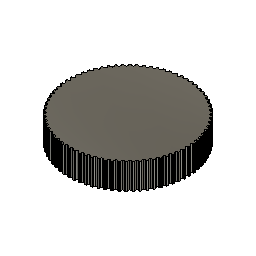
gear_74z (Autodesk Fusion 360 design; units mm, degrees)
Autodesk Fusion 360 part; units mm, degrees
sketch "Sketch1" plane through (0, 0, 0) normal (0, 0, 1) x (1, 0, 0) in component "gt2 pulley"
  circle A0 centre (0, 0) radius 23.5549 construction
  circle A1 centre (0, 0) radius 22.5509 construction
  line L0 (0, 0) -> (0, 23.5549) construction
  line L1 (0, 0) -> (0.9997, 23.5337) construction
  line L2 (0, 0) -> (1.4052, 23.513) construction
  circle A2 centre (0, 0) radius 23.3009 construction
  arc A3 (0.3946, 23.164) -> (0.47, 22.8677) centre (1.3901, 23.2594) ccw
  circle A4 centre (0, 0) radius 23.1509 construction
  arc A5 (0.2469, 23.2996) -> (0, 23.3009) centre (0, 0) ccw
  arc A6 (0.3946, 23.164) -> (0.2469, 23.2996) centre (0.2453, 23.1496) ccw
  arc A7 (0.47, 22.8677) -> (0.9571, 22.5306) centre (0.9806, 23.0851) ccw
  arc A8 (0, 23.3009) -> (-0.2469, 23.2996) centre (0, 0) ccw
  arc A9 (-0.2469, 23.2996) -> (-0.3946, 23.164) centre (-0.2453, 23.1496) ccw
  arc A10 (-0.47, 22.8677) -> (-0.3946, 23.164) centre (-1.3901, 23.2594) ccw
  arc A11 (-0.9573, 22.5306) -> (-0.47, 22.8677) centre (-0.9806, 23.0851) ccw
  arc A12 (0.9571, 22.5306) -> (-0.9571, 22.5306) centre (0, 0) ccw
  point P0 (1.3901, 23.2594)
  point P1 (0, 23.3009)
  dimension "d18" = 47.1099
  dimension "d19" = 2.432
  dimension "d22" = 1.004
  dimension "d24" = 0.75
  dimension "d26" = 1
  dimension "d27" = 0.15
  dimension "d28" = 0.15
  dimension "d47" = 0.555
  dimension "d52" = 3.812
  constraint coincident A0.centre A1.centre
  constraint coincident A0 L0.end
  constraint vertical L0
  constraint coincident A0 L1.end
  constraint coincident A0 L2.end
  constraint concentric A1 A2
  constraint coincident A1 A7.end
  constraint coincident L1 A7.end
  constraint coincident A2 P0
  constraint coincident L2 P0
  constraint coincident P0 A3.centre
  constraint coincident A2 P1
  constraint coincident L0 P1
  constraint concentric A2 A4
  constraint coincident P1 A5.end
  constraint coincident A4 A6.centre
  constraint coincident A3.start A6.start
  constraint tangent A3 A6
  constraint tangent A3 A7
  constraint symmetric L0 A7.end A12.end
  constraint symmetric L0 A3.start A9.end
  constraint symmetric L0 A3.end A10.start
  constraint symmetric L0 A3 A10
  constraint symmetric L0 A5.start A8.end
  constraint symmetric L0 P1 A5.end
  constraint symmetric L0 A5 A8
  constraint symmetric L0 A6 A9
  constraint symmetric L0 A7 A11
  constraint coincident A1 A11.start
  constraint tangent A1 A7
  constraint coincident L1 A7.centre
  measures "d18" diameter of A0
  measures "d19" angle of L0 L1
  measures "d22" distance of A0 A1
  measures "d24" distance of A1 A2
  measures "d26" radius of A3
  measures "d27" distance of A2 A4
  measures "d28" radius of A6
  measures "d47" radius of A7
extrude "Extrude1" add sketch "Sketch1" along normal blind 10 makes body 1
pattern_circular "C-Pattern1" count 74 over 360 about axis through (0, 0, 1.75) along (0, 0, 1) of bodies 1 makes body 2 at (-2.6534, 22.3943, 6.6667) makes body 3 at (-3.9161, 22.2083, 6.6667) makes body 4 at (-6.3999, 21.6237, 6.6667) makes body 5 at (-8.2107, 21.0031, 6.6667) makes body 6 at (-9.3857, 20.5049, 6.6667) makes body 7 at (-11.6421, 19.3133, 6.6667) makes body 8 at (-13.0652, 18.3805, 6.6667) makes body 9 at (-14.5769, 17.2063, 6.6667) makes body 10 at (-16.133, 15.7566, 6.6667) makes body 11 at (-16.4273, 15.4496, 3.3333) makes body 12 at (-18.5638, 12.8035, 6.6667) makes body 13 at (-19.2584, 11.7328, 6.6667) makes body 14 at (-19.7902, 10.8117, 6.6667) makes body 15 at (-21.191, 7.7127, 6.6667) makes body 16 at (-21.5934, 6.5015, 6.6667) makes body 17 at (-22.067, 4.6468, 6.6667) makes body 18 at (-22.3816, 2.7587, 6.6667) makes body 19 at (-22.5259, 1.0632, 6.6667) makes body 20 at (-22.5258, -1.0635, 6.6667) makes body 21 at (-22.3815, -2.7589, 6.6667) makes body 22 at (-22.0221, -4.8551, 6.6667) makes body 23 at (-21.531, -6.7052, 6.6667) makes body 24 at (-21.1909, -7.7129, 3.3333) makes body 25 at (-19.7901, -10.812, 6.6667) makes body 26 at (-19.5826, -11.1832, 3.3333) makes body 27 at (-18.5637, -12.8037, 3.3333) makes body 28 at (-17.411, -14.3319, 3.3333) makes body 29 at (-15.5268, -16.3543, 6.6667) makes body 30 at (-14.7384, -17.0682, 3.3333) makes body 31 at (-12.5396, -18.7431, 6.6667) makes body 32 at (-10.5304, -19.9413, 6.6667) makes body 33 at (-9.9621, -20.2312, 6.6667) makes body 34 at (-7.4121, -21.298, 6.6667) makes body 35 at (-4.9585, -21.999, 6.6667) makes body 36 at (-3.075, -22.3403, 6.6667) makes body 37 at (-1.1694, -22.5206, 6.6667) makes body 38 at (0.7447, -22.5386, 6.6667) makes body 39 at (2.6534, -22.3943, 6.6667) makes body 40 at (3.9161, -22.2083, 6.6667) makes body 41 at (5.7854, -21.7962, 6.6667) makes body 42 at (6.8066, -21.4992, 3.3333) makes body 43 at (9.3857, -20.5049, 6.6667) makes body 44 at (11.0908, -19.6351, 6.6667) makes body 45 at (12.7161, -18.6238, 6.6667) makes body 46 at (14.5769, -17.2063, 6.6667) makes body 47 at (16.133, -15.7566, 6.6667) makes body 48 at (16.4273, -15.4496, 3.3333) makes body 49 at (18.5638, -12.8035, 6.6667) makes body 50 at (18.802, -12.4511, 3.3333) makes body 51 at (19.7902, -10.8117, 3.3333) makes body 52 at (21.191, -7.7127, 6.6667) makes body 53 at (21.5934, -6.5015, 6.6667) makes body 54 at (22.1897, -4.0204, 6.6667) makes body 55 at (22.3816, -2.7587, 6.6667) makes body 56 at (22.5499, -0.2125, 6.6667) makes body 57 at (22.5258, 1.0635, 6.6667) makes body 58 at (22.2615, 3.6015, 6.6667) makes body 59 at (22.0221, 4.8551, 6.6667) makes body 60 at (21.531, 6.7052, 6.6667) makes body 61 at (20.8848, 8.507, 6.6667) makes body 62 at (20.0881, 10.2475, 6.6667) makes body 63 at (19.5826, 11.1832, 3.3333) makes body 64 at (18.0673, 13.495, 6.6667) makes body 65 at (17.411, 14.3319, 3.3333) makes body 66 at (15.0577, 16.7872, 6.6667) makes body 67 at (14.0839, 17.6122, 6.6667) makes body 68 at (12.5396, 18.7431, 6.6667) makes body 69 at (11.6419, 19.3135, 3.3333) makes body 70 at (9.9621, 20.2312, 6.6667) makes body 71 at (6.8063, 21.4993, 6.6667) makes body 72 at (4.9585, 21.999, 6.6667) makes body 73 at (3.075, 22.3403, 6.6667) makes body 74 at (1.1694, 22.5206, 6.6667)
sketch "Sketch2" plane through (0, 0, 10) normal (0, 0, 1) x (-1, 0, 0)
  arc A0 (-9.9009, -20.9451) -> (-9.8221, -21.1296) centre (-9.7589, -20.9936) ccw
  arc A1 (-9.8221, -21.1296) -> (-9.3722, -21.333) centre (0, 0) ccw
  arc A2 (-9.3722, -21.333) -> (-9.1816, -21.2702) centre (-9.3118, -21.1957) ccw
  arc A3 (-8.991, -21.0313) -> (-9.1816, -21.2702) centre (-8.3139, -21.7672) ccw
  arc A4 (-8.4083, -20.9248) -> (-8.991, -21.0313) centre (-8.6152, -21.4397) ccw
  arc A5 (-10.1525, -20.1363) -> (-8.4083, -20.9248) centre (0, 0) ccw
  arc A6 (-9.8475, -20.6441) -> (-10.1525, -20.1363) centre (-10.4024, -20.6319) ccw
  arc A7 (-9.9009, -20.9451) -> (-9.8475, -20.6441) centre (-10.8473, -20.6221) ccw
  circle A8 centre (0, 0) radius 22.5509
  constraint coincident A1.centre A5.centre
extrude "Extrude2" add sketch "Sketch2" against normal blind 10 contours A5 A8 bodies 1 2 3 4 5 6 7 8 9 10 11 12 13 14 15 16 17 18 19 20 21 22 23 24 25 26 27 28 29 30 31 32 33 34 35 36 37 38 39 40 41 42 43 44 45 46 47 48 49 50 51 52 53 54 55 56 57 58 59 60 61 62 63 64 65 66 67 68 69 70 71 72 73 74
extrude "Extrude4" [suppressed] in component "gt2 pulley"
pattern_circular "C-Pattern7" [suppressed] in component "gt2 pulley"
extrude "Extrude3" [suppressed] in component "gt2 pulley"
pattern_circular "C-Pattern6" [suppressed] in component "gt2 pulley"
extrude "Extrude2'" [suppressed] in component "gt2 pulley"
pattern_circular "C-Pattern5" [suppressed] in component "gt2 pulley"
extrude "Extrude1'" [suppressed] in component "gt2 pulley"
pattern_circular "C-Pattern4" [suppressed] in component "gt2 pulley"
pattern_circular "C-Pattern3" [suppressed] in component "gt2 pulley"
pattern_circular "C-Pattern2" [suppressed] in component "gt2 pulley"
pattern_circular "C-Pattern1'" [suppressed] in component "gt2 pulley"
copy_body "Body->Comp1" [suppressed] in component "Component"
copy_body "Body->Comp2" [suppressed] in component "Component'"
copy_body "Body->Comp3" [suppressed] in component "Component''"
copy_body "Body->Comp4" [suppressed] in component "Component'''"
copy_body "Body->Comp5" [suppressed] in component "Component''''"
copy_body "Body->Comp6" [suppressed] in component "Component'''''"
copy_body "Body->Comp7" [suppressed] in component "Component''''''"
copy_body "Body->Comp8" [suppressed] in component "Component'''''''"
copy_body "Body->Comp9" [suppressed] in component "Component''''''''"
copy_body "Body->Comp10" [suppressed] in component "Component'''''''''"
copy_body "Body->Comp11" [suppressed] in component "Component''''''''''"
copy_body "Body->Comp12" [suppressed] in component "Component'''''''''''"
copy_body "Body->Comp13" [suppressed] in component "Component''''''''''''"
copy_body "Body->Comp14" [suppressed] in component "Component'''''''''''''"
copy_body "Body->Comp15" [suppressed] in component "Component''''''''''''''"
copy_body "Body->Comp16" [suppressed] in component "Component'''''''''''''''"
copy_body "Body->Comp17" [suppressed] in component "Component''''''''''''''''"
copy_body "Body->Comp18" [suppressed] in component "Component'''''''''''''''''"
copy_body "Body->Comp19" [suppressed] in component "Component''''''''''''''''''"
copy_body "Body->Comp20" [suppressed] in component "Component'''''''''''''''''''"
component "gt2 pulley" placed x (1, 0, 0) y (0, 1, 0) z (0, 0, 1) at (0, 0, 0)
equation "NumTeeth = 74" comment "min 20"
equation "ToothPitch = 2 mm"
equation "PullyDia = NumTeeth * ToothPitch / PI"
equation "ToothAng = ( ( 360 / NumTeeth ) * 1 deg )"
equation "TransOffsetAngle = ToothAng * 0.2"
equation "Sholulder_Radius = 0.15 mm"
equation "Root_Radius = 0.555 mm"
equation "TransRadius = 1 mm"
equation "ToolHeight = 0.75 mm"
equation "PLD = 0.254 mm"
equation "d18 = PullyDia"
equation "d19 = ToothAng / 2"
equation "d22 = PLD + ToolHeight"
equation "d24 = ToolHeight"
equation "d26 = TransRadius"
equation "d27 = Sholulder_Radius"
equation "d31 = NumTeeth"
equation "d33 = NumTeeth"
equation "d35 = NumTeeth"
equation "d37 = NumTeeth"
equation "d41 = NumTeeth"
equation "d45 = NumTeeth"
equation "d47 = Root_Radius"
equation "d50 = NumTeeth"
